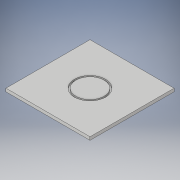
# Autodesk Inventor part: bottom
Saved by Autodesk Inventor 2019 (Build 230136000, 136)
## iProperties
Created: 2018-10-31
Part Number: bottom
Material: Generic
Document SubType Name: Modeling
Designer: 2003189
Density: 1 g/cm^3
Appearance: Default
Author: 2003189
Autodesk Inventor part; units mm, degrees
ref_plane "YZ Plane" through (0, 0, 0) normal (1, 0, 0) x (0, 1, 0)
ref_plane "XZ Plane" through (0, 0, 0) normal (0, 1, 0) x (-1, 0, 0)
ref_plane "XY Plane" through (0, 0, 0) normal (0, 0, 1) x (1, 0, 0)
sketch "Sketch1" plane through (0, 0, 0) normal (0, 1, 0) x (-1, 0, 0)
  line L0 (0, 0) -> (-342.9, 0)
  line L1 (-342.9, 0) -> (-342.9, -342.9)
  line L2 (-342.9, -342.9) -> (0, -342.9)
  line L3 (0, -342.9) -> (0, 0)
  dimension "d0" = 342.9
  dimension "d1" = 342.9
  constraints: 8 end point, 2 parallel, 1 horizontal, 1 perpendicular
  measures "d0" distance of L2.end L1.end
  measures "d1" distance of L1.end L0.end
extrude "Extrusion1" add sketch "Sketch1" along normal blind 12.7
sketch "Sketch2" plane through (0, 12.7, 0) normal (0, 1, 0) x (1, 0, 0)
  line L0 (0, 0) -> (342.9, 0) projected
  line L1 (171.45, 0) -> (171.45, 342.9)
  line L2 (342.9, 342.9) -> (0, 342.9) projected
  circle A0 centre (171.45, 171.45) radius 57.15
  circle A1 centre (171.45, 171.45) radius 63.5
  dimension "d4" = 114.3
  dimension "d5" = 6.35
  constraints: 3 midpoint, 2 centre point, 2 end point
  measures "d4" diameter of A0
  measures "d5" radial gap between concentric circles of A0 A1
extrude "Extrusion2" cut sketch "Sketch2" against normal blind 6.35 contours A1 L1 A0 | L1 A0 A1
body "Solid1"
